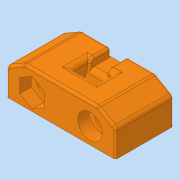
# Autodesk Inventor part: CarriageImproved
Saved by Autodesk Inventor 2017.3 (Build 213256000, 256)
## iProperties
Created: 2018-04-03
Part Number: CarriageImproved
Material: ABS Plastic
Document SubType Name: Modeling
Designer: Derek Wider
Density: 1.06 g/cm^3
Appearance: Orange
Author: Derek Wider
Autodesk Inventor part; units mm, degrees
ref_plane "YZ Plane" through (0, 0, 0) normal (1, 0, 0) x (0, 1, 0)
sketch "Sketch1" plane through (0, 0, 0) normal (0, 0, 1) x (1, 0, 0)
  circle A0 centre (0, 0) radius 3.3655
  circle A1 centre (0, 0) radius 1.905
  circle A2 centre (-15.875, 0) radius 1.905
  line L0 (-15.875, -3.8861) -> (-19.2405, -1.9431)
  line L1 (-19.2405, -1.9431) -> (-19.2405, 1.9431)
  line L2 (-19.2405, 1.9431) -> (-15.875, 3.8861)
  line L3 (-15.875, 3.8861) -> (-12.5095, 1.9431)
  line L4 (-12.5095, 1.9431) -> (-12.5095, -1.9431)
  line L5 (-12.5095, -1.9431) -> (-15.875, -3.8861)
  line L6 (-22.86, 5.715) -> (6.985, 5.715)
  line L7 (6.985, 5.715) -> (6.985, -4.445)
  line L8 (6.985, -4.445) -> (-22.86, -4.445)
  line L9 (-22.86, -4.445) -> (-22.86, 5.715)
  dimension "d0" = 6.731
  dimension "d1" = 3.81
  dimension "d2" = 3.81
  dimension "d3" = 6.731
  dimension "d4" = 15.875
  dimension "d5" = 10.16
  dimension "d6" = 29.845
  dimension "d30" = 4.445
  dimension "d31" = 6.985
  constraints: 20 end point, 3 centre point, 3 coincident, 2 parallel, 1 horizontal, 1 horizontal alignment, 1 perpendicular, 1 vertical, 13 other
  measures "d0" diameter of A0
  measures "d1" diameter of A1
  measures "d2" diameter of A2
  measures "d3" distance between parallel lines of L4 L1
  measures "d4" distance of A2.centre point (0, 0)
  measures "d5" distance of L6.end L7.end
  measures "d6" distance of L7.end L8.end
  measures "d30" vertical distance of L7.end point (0, 0)
  measures "d31" distance from line of L7 point (0, 0)
extrude "Extrusion1" add sketch "Sketch1" along normal blind 15.875 contours L6 L7 L8 L9
ref_plane "Work Plane1" through (0, 0, 3.175) normal (0, 0, -1) x (-1, 0, 0)
sketch "Sketch2" plane through (0, 0, 3.175) normal (0, 0, -1) x (-1, 0, 0)
  circle A0 centre (0, 0) radius 1.905 projected
  circle A1 centre (0, 0) radius 3.3655 projected
  circle A2 centre (15.875, 0) radius 1.905 projected
  line L0 (19.2405, 1.9431) -> (19.2405, -1.9431) projected
  line L1 (19.2405, -1.9431) -> (15.875, -3.8861) projected
  line L2 (15.875, -3.8861) -> (12.5095, -1.9431) projected
  line L3 (12.5095, -1.9431) -> (12.5095, 1.9431) projected
  line L4 (12.5095, 1.9431) -> (15.875, 3.8861) projected
  line L5 (15.875, 3.8861) -> (19.2405, 1.9431) projected
  circle A3 centre (0, 0) radius 3.3655 projected
  line L6 (22.86, 5.715) -> (-6.985, 5.715) projected
  line L7 (-6.985, 5.715) -> (-6.985, -4.445) projected
  line L8 (-6.985, -4.445) -> (22.86, -4.445) projected
  line L9 (22.86, -4.445) -> (22.86, 5.715) projected
extrude "Extrusion2" add sketch "Sketch2" against normal blind 9.525 contours A1 | L0 L1 L2 L3 L4 L5
ref_plane "Work Plane2" through (0, 0, 7.9375) normal (0, 0, -1) x (-1, 0, 0)
sketch "Sketch4" plane through (0, 0, 7.9375) normal (0, 0, -1) x (-1, 0, 0)
  circle A0 centre (0, 0) radius 1.905 construction
  circle A1 centre (15.875, 0) radius 1.905 construction
  line L0 (-6.985, -4.445) -> (-6.985, 5.715) construction
  line L1 (-6.985, 5.715) -> (22.86, 5.715) construction
  line L2 (22.86, 5.715) -> (22.86, -4.445) construction
  line L3 (22.86, -4.445) -> (-6.985, -4.445) construction
  line L4 (22.86, 5.715) -> (-6.985, 5.715) projected
  line L5 (-6.985, -4.445) -> (22.86, -4.445) projected
  arc A2 (10.795, 5.715) -> (14.351, -4.445) centre (26.0305, 5.3451) ccw
  line L6 (10.795, 5.715) -> (3.81, 5.715)
  line L7 (3.81, 5.715) -> (3.81, -4.445)
  line L8 (3.81, -4.445) -> (14.351, -4.445)
  dimension "d14" = 15.24
  dimension "d15" = 12.065
  dimension "d16" = 8.509
  dimension "d17" = 10.795
  constraints: 6 end point, 4 point on line, 2 perpendicular, 2 point on circle, 1 centre point
  measures "d14" radius of A2
  measures "d15" distance of L1.end L6.start
  measures "d16" distance of L2.end L8.end
  measures "d17" distance between parallel lines of L0 L7
extrude "Extrusion3" cut sketch "Sketch4" along normal mid plane 4.445
fillet "Fillet4" radius 1.27 4 edges at (-7.3025, 5.715, 5.715) (-7.3025, 5.715, 10.16) (-3.81, 5.715, 7.9375) (-10.795, 5.715, 7.9375)
chamfer "Chamfer1" distance 4.826 distance2 2.794 1 edges at (-22.86, 5.715, 7.9375) measured on face at (-19.2698, 5.715, 6.7733)
chamfer "Chamfer2" distance 4.826 distance2 2.794 1 edges at (6.985, 5.715, 7.9375) measured on face at (3.81, 5.715, 9.1017)
fillet "Fillet5" radius 1.27 4 edges at (-18.034, 5.715, 7.9375) (-22.86, 2.921, 7.9375) (2.159, 5.715, 7.9375) (6.985, 2.921, 7.9375)
fillet "Fillet6" radius 0.635 18 edges at (-18.0223, 5.6715, 15.875) (-20.2778, 4.416, 15.875) (-22.6902, 2.8231, 15.875) (-22.86, -1.1281, 15.875) (2.1473, 5.6715, 15.875) (4.4028, 4.416, 15.875) (6.8152, 2.8231, 15.875) (6.985, -1.1281, 15.875) (-7.9375, 5.715, 15.875) (2.1473, 5.6715, 0) (4.4028, 4.416, 0) (6.8152, 2.8231, 0) (6.985, -1.1281, 0) (-18.0223, 5.6715, 0) (-20.2778, 4.416, 0) (-22.6902, 2.8231, 0) (-22.86, -1.1281, 0) (-7.9375, 5.715, 0)
sketch "Sketch5" plane through (0, 0, 0) normal (0, 0, -1) x (-1, 0, 0)
  line L0 (5.715, 5.715) -> (10.16, 5.715)
  line L1 (10.16, 5.715) -> (10.16, 3.429)
  line L2 (10.16, 3.429) -> (5.715, 3.429)
  line L3 (5.715, 3.429) -> (5.715, 5.715)
  circle A0 centre (15.875, 0) radius 1.905 construction
  circle A1 centre (0, 0) radius 1.905 construction
  line L4 (0, 0) -> (15.875, 0) construction
  line L5 (17.6929, 5.715) -> (-1.8179, 5.715) construction
  point P0 (7.9375, 3.429)
  point P1 (7.9375, 0)
  dimension "d32" = 4.445
  dimension "d33" = 2.286
  constraints: 10 end point, 2 horizontal, 2 midpoint, 2 parallel, 1 perpendicular, 1 point on line, 1 vertical alignment
  measures "d32" distance of L0.start L0.end
  measures "d33" distance of L2.end L0.start
extrude "Extrusion4" cut sketch "Sketch5" against normal up to surface (5.715 mm away)
fillet "Fillet7" radius 0.635 10 edges at (-5.715, 5.529, 0.186) (-5.715, 5.715, 2.54) (-5.715, 5.343, 5.343) (-5.715, 3.937, 5.715) (-5.715, 4.2545, 0) (-10.16, 5.529, 0.186) (-10.16, 5.715, 2.54) (-10.16, 5.343, 5.343) (-10.16, 3.937, 5.715) (-10.16, 4.2545, 0)
fillet "Fillet8" radius 1.27 1 edges at (-7.9375, 3.429, 5.715)
equation "\"d31\" = -0.5 * d4 + 0.5 * d6"
body "Solid1"
